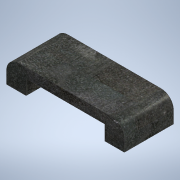
# Autodesk Inventor part: newsteelhandle
Saved by Autodesk Inventor 2020.1 (Build 241239000, 239)
## iProperties
Created: 2021-08-04
Part Number: newsteelhandle
Material: Steel
Document SubType Name: Modeling
Designer: Caleb
Density: 7.85 g/cm^3
Appearance: Plate
Author: Caleb
Autodesk Inventor part; units mm, degrees
ref_plane "YZ Plane" through (0, 0, 0) normal (1, 0, 0) x (0, 1, 0)
ref_plane "XZ Plane" through (0, 0, 0) normal (0, 1, 0) x (-1, 0, 0)
ref_plane "XY Plane" through (0, 0, 0) normal (0, 0, 1) x (1, 0, 0)
sketch "Sketch1" plane through (0, 0, 0) normal (0, 1, 0) x (-1, 0, 0)
  line L0 (60, 25) -> (-60, 25)
  line L1 (-60, 25) -> (-60, -25)
  line L2 (-60, -25) -> (60, -25)
  line L3 (60, -25) -> (60, 25)
  point P0 (0, 0)
  constraints: 8 end point, 2 parallel, 1 horizontal, 1 perpendicular
extrude "Extrusion1" add sketch "Sketch1" along normal mid plane 25
sketch "Sketch2" plane through (-60, 12.5, 25) normal (0, 0, 1) x (1, 0, 0)
  line L0 (0, -25) -> (120, -25) projected
  line L1 (60, -25) -> (20, -25)
  line L2 (20, -25) -> (20, -10)
  line L3 (20, -10) -> (100, -10)
  line L4 (100, -10) -> (100, -25)
  line L5 (100, -25) -> (60, -25)
  point P0 (60, -12.5)
  dimension "d5" = 15
  dimension "d6" = 80
  constraints: 10 end point, 3 perpendicular, 2 point on line, 1 collinear, 1 midpoint
  measures "d5" distance of L1.end L2.end
  measures "d6" distance of L2.end L3.end
extrude "Extrusion2" cut sketch "Sketch2" against normal through all
fillet "Fillet1" radius 12.5 2 edges at (60, 12.5, 0) (-60, 12.5, 0)
sketch "Sketch3" plane through (0, -12.5, 0) normal (0, -1, 0) x (1, 0, 0)
  line L0 (-60, 25) -> (-60, -25) projected
  line L1 (60, -25) -> (60, 25) projected
  point P0 (0, 0)
  point P1 (-50, 0)
  point P2 (50, 0)
hole "Hole1" at (-50, -12.5, 0) at (50, -12.5, 0) direction (0, 1, 0) diameter 3 depth 0.5 tip angle 118
body "Solid1"
